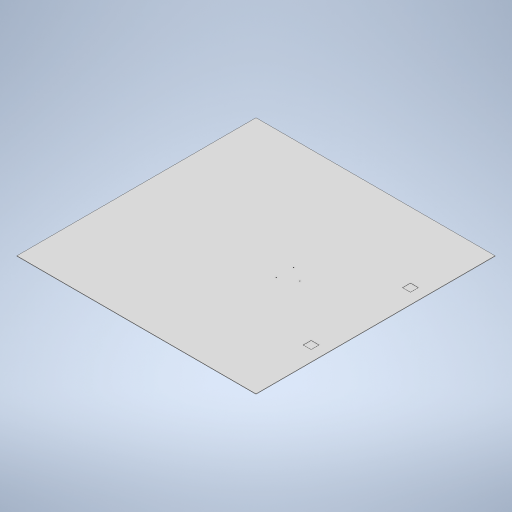
# Autodesk Inventor part: Piso
Saved by Autodesk Inventor 2024 (Build 280153000, 153)
## iProperties
Created: 2023-04-22
Part Number: Piso
Material: Genérico
Document SubType Name: Modeling
Designer: javie
Density: 1 g/cm^3
Appearance: Valor por defecto
Author: javie
Autodesk Inventor part; units mm, degrees
ref_plane "YZ Plane" through (0, 0, 0) normal (1, 0, 0) x (0, 1, 0)
ref_plane "XZ Plane" through (0, 0, 0) normal (0, 1, 0) x (-1, 0, 0)
ref_plane "XY Plane" through (0, 0, 0) normal (0, 0, 1) x (1, 0, 0)
sketch "Boceto1" plane through (0, 0, 0) normal (0, 1, 0) x (-1, 0, 0)
  line L0 (3000, 3000) -> (-3000, 3000)
  line L1 (-3000, 3000) -> (-3000, -3000)
  line L2 (-3000, -3000) -> (3000, -3000)
  line L3 (3000, -3000) -> (3000, 3000)
  point P0 (0, 0)
  dimension "d0" = 6000
  dimension "d1" = 6000
  constraints: 8 end point, 2 parallel, 1 horizontal, 1 perpendicular
  measures "d0" distance of L2.end L1.end
  measures "d1" distance of L1.end L0.end
extrude "Extrusión1" add sketch "Boceto1" along normal blind 10
sketch "Boceto2" plane through (0, 10, 0) normal (0, 1, 0) x (1, 0, 0)
  circle A0 centre (1100, 0) radius 9.25
  line L0 (3000, -3000) -> (3000, 3000) projected
  circle A1 centre (725, 0) radius 9.25
  circle A2 centre (725, -216.5) radius 9.25
  circle A3 centre (725, 216.5) radius 9.25
  point P0 (0, 0)
  dimension "d4" = 18.5
  dimension "d5" = 1900
  dimension "d6" = 18.5
  dimension "d7" = 375
  dimension "d8" = 18.5
  dimension "d9" = 18.5
  dimension "d10" = 216.5
  dimension "d14" = 375
  constraints: 4 centre point
  measures "d4" diameter of A0
  measures "d5" distance from line of A0.centre L0
  measures "d6" diameter of A1
  measures "d7" distance of A1.centre A0.centre
  measures "d8" diameter of A2
  measures "d9" diameter of A3
  measures "d10" distance of A2.centre A1.centre
  measures "d14" horizontal distance of A0.centre A3.centre
extrude "Extrusión2" cut sketch "Boceto2" against normal blind 10 contours A0 | A2 | A3
sketch "Boceto3" plane through (0, 10, 0) normal (0, 1, 0) x (1, 0, 0)
  line L0 (2730, -1145.997) -> (2530, -1145.997)
  line L1 (2530, -1145.997) -> (2530, -1345.997)
  line L2 (2530, -1345.997) -> (2730, -1345.997)
  line L3 (2730, -1345.997) -> (2730, -1145.997)
  line L4 (2730, 1345.9966) -> (2530, 1345.9966)
  line L5 (2530, 1345.9966) -> (2530, 1145.9966)
  line L6 (2530, 1145.9966) -> (2730, 1145.9966)
  line L7 (2730, 1145.9966) -> (2730, 1345.9966)
  circle A0 centre (1100, 0) radius 9.25 projected
  point P0 (0, 0)
  point P1 (2630, -1345.997)
  point P2 (2630, 1345.9966)
  point P3 (2730, -1245.997)
  dimension "d15" = 200
  dimension "d16" = 200
  dimension "d17" = 200
  dimension "d18" = 2691.9936
  dimension "d19" = 1345.997
  dimension "d21" = 1630
  constraints: 16 end point, 4 parallel, 3 midpoint, 2 horizontal, 2 perpendicular, 2 point on line
  measures "d15" distance of L2.end L1.end
  measures "d16" distance of L1.end L0.end
  measures "d17" distance of L5.end L4.end
  measures "d18" distance of point (2630, -1345.997) point (2630, 1345.997)
  measures "d19" vertical distance of point (0, 0) point (2630, -1345.997)
  measures "d21" horizontal distance of A0.centre point (2730, -1245.997)
extrude "Extrusión3" cut sketch "Boceto3" against normal blind 4 contours L3 L2 L1 L0 | L7 L6 L5 L4
